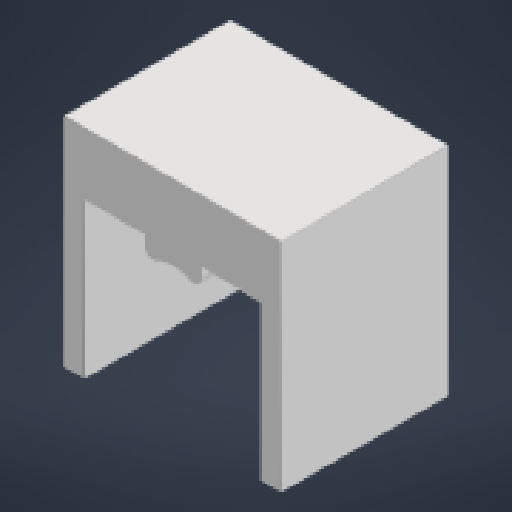
# Autodesk Inventor part: PRINTED resin filament path
Saved by Autodesk Inventor 2024 (Build 280153000, 153)
## iProperties
Created: 2024-07-28
Part Number: PRINTED resin filament path
Material: Generic
Document SubType Name: Modeling
Designer: mateu
Density: 1 g/cm^3
Appearance: Default
Author: mateu
Autodesk Inventor part; units mm, degrees
ref_plane "YZ Plane" through (0, 0, 0) normal (1, 0, 0) x (0, 1, 0)
ref_plane "XZ Plane" through (0, 0, 0) normal (0, 1, 0) x (-1, 0, 0)
ref_plane "XY Plane" through (0, 0, 0) normal (0, 0, 1) x (1, 0, 0)
sketch "Sketch1" plane through (0, 0, 0) normal (0, 0, 1) x (1, 0, 0)
  line L0 (3.45, 2.4) -> (3.45, 4.7)
  line L1 (3.45, 4.7) -> (1.9, 4.7)
  line L2 (1.9, 2.4) -> (1.9, 4.7)
  line L3 (0, 2.4) -> (0, 4.7)
  line L4 (0, 4.7) -> (-1.55, 4.7)
  line L5 (-1.55, 2.4) -> (-1.55, 4.7)
  line L6 (-1.55, 0) -> (-1.55, 2.4)
  line L7 (3.45, 0) -> (3.45, 2.4)
  circle A0 centre (0.95, 3.425) radius 1
  line L8 (4.45, -0.05) -> (4.45, 6.95)
  line L9 (4.45, 6.95) -> (-2.55, 6.95)
  line L10 (-2.55, -0.05) -> (-2.55, 6.95)
  line L11 (-2.25, 6.65) -> (4.15, 6.65)
  line L12 (4.15, 6.65) -> (4.15, 0.25)
  line L13 (4.15, 0.25) -> (-2.25, 0.25)
  line L14 (-2.25, 0.25) -> (-2.25, 6.65)
  line L15 (1.8, 2.4) -> (1.8, 4.8)
  line L16 (1.8, 4.8) -> (3.55, 4.8)
  line L17 (3.55, 4.8) -> (3.55, 2.4)
  line L18 (3.55, 2.4) -> (3.55, 0)
  line L19 (-1.65, 0) -> (-1.65, 2.4)
  line L20 (-1.65, 2.4) -> (-1.65, 4.8)
  line L21 (-1.65, 4.8) -> (0.1, 4.8)
  line L22 (0.1, 4.8) -> (0.1, 2.4)
  circle A1 centre (0.95, 3.425) radius 0.875
  circle A2 centre (0.95, 3.425) radius 1
  circle A3 centre (1.55, 4.521586) radius 0.25
  circle A4 centre (0.35, 4.521586) radius 0.25
  line L23 (4.45, -0.05) -> (-2.55, -0.05)
  point P0 (0, 0)
  point P1 (-1.65, 0.25)
  point P2 (0.1, 4.521586)
  point P3 (0.47, 4.302268)
  point P4 (1.43, 4.302268)
  point P5 (1.8, 4.521586)
  point P6 (3.55, 0.25)
  dimension "d0" = 0.3
  dimension "d1" = 0.1
  dimension "d2" = 0.1
  dimension "d3" = 2
  dimension "d4" = 0.5
  constraints: 24 end point, 4 tangent, 3 centre point, 1 coincident, 1 equal radius, 7 other
  measures "d0" distance between parallel lines of L9 L11
  measures "d1" distance between parallel lines of L0 L17
  measures "d2" distance between parallel lines of L4 L21
  measures "d3" diameter of A2
  measures "d4" diameter of A3
extrude "Extrusion1" add sketch "Sketch1" against normal blind 4.9 contours L18 L17 L16 L15 A3 A0 A4 L22 L21 L20 L19 L13 L14 L11 L12 | A3 | A4
sketch "Sketch2" plane through (0, 0, -4.9) normal (0, 0, -1) x (-1, 0, 0)
  line L0 (-3.55, 0.25) -> (-4.15, 0.25)
  line L1 (-3.55, 0.25) -> (-3.55, 1.25)
  line L2 (-3.55, 4.8) -> (-3.55, 0.25)
  line L3 (-3.55, 1.25) -> (1.739721, 1.25)
  line L4 (2.25, 6.65) -> (-4.15, 6.65)
  line L5 (-4.15, 6.65) -> (-4.15, 0.25)
  line L6 (-4.15, 0.25) -> (-3.55, 0.25)
  line L7 (-3.55, 0.25) -> (-3.55, 4.8)
  line L8 (-3.55, 4.8) -> (-1.8, 4.8)
  line L9 (-1.8, 4.8) -> (-1.8, 4.521586)
  arc A0 (-1.8, 4.521586) -> (-1.43, 4.302268) centre (-1.55, 4.521586) ccw
  arc A1 (-0.47, 4.302268) -> (-1.43, 4.302268) centre (-0.95, 3.425) ccw
  arc A2 (-0.47, 4.302268) -> (-0.1, 4.521586) centre (-0.35, 4.521586) ccw
  line L10 (-0.1, 4.521586) -> (-0.1, 4.8)
  line L11 (-0.1, 4.8) -> (1.65, 4.8)
  line L12 (1.65, 4.8) -> (1.65, 0.25)
  line L13 (1.65, 0.25) -> (2.25, 0.25)
  line L14 (2.25, 0.25) -> (2.25, 6.65)
  circle A3 centre (-0.95, 3.425) radius 1
  point P0 (0, 0)
  point P1 (1.65, 1.25)
  point P2 (-0.47, 4.302268)
  dimension "d8" = 1
  constraints: 4 end point, 1 centre point, 1 coincident, 1 concentric, 1 perpendicular, 1 point on line
  measures "d8" distance of L0.start L1.end
extrude "Extrusion2" add sketch "Sketch2" against normal blind 0.8 contours L2 L8 L9 A0 A3 A2 L10 L11 L12 L3
chamfer "Chamfer1" distance 0.5 angle 20 1 edges at (0.95, 2.425, -4.1) measured on face at (0.95, 2.425, -4.6)
sketch "Sketch3" plane through (0, 0, 0) normal (0, 0, 1) x (1, 0, 0)
  arc A0 (0.189544, 4.329873) -> (1.710456, 4.329873) centre (0.95, 3.425) ccw
  arc A1 (0.1, 4.521586) -> (0.189544, 4.329873) centre (0.35, 4.521586) ccw
  line L0 (0.1, 4.8) -> (0.1, 4.521586)
  line L1 (-1.65, 4.8) -> (0.1, 4.8)
  line L2 (-1.65, 1.25) -> (-1.65, 4.8)
  line L3 (-1.65, 1.25) -> (3.55, 1.25)
  line L4 (3.55, 4.8) -> (3.55, 1.25)
  line L5 (1.8, 4.8) -> (3.55, 4.8)
  line L6 (1.8, 4.521586) -> (1.8, 4.8)
  arc A2 (1.710456, 4.329873) -> (1.8, 4.521586) centre (1.55, 4.521586) ccw
  spline S0 degree 7 poles (1.710456, 4.329873) (1.702909, 4.323556) (1.695037, 4.317557) (1.686841, 4.311886) (1.678321, 4.306557) (1.669477, 4.301587) (1.660303, 4.296994) (1.636622, 4.286561) (1.621727, 4.281222) (1.606064, 4.276852) (1.589598, 4.273563) (1.572312, 4.271515) (1.554218, 4.270908) (1.520976, 4.272859) (1.506137, 4.274699) (1.490907, 4.277659) (1.475421, 4.281858) (1.459899, 4.287391) (1.444641, 4.294258) (1.43, 4.302268) knots 0 0 0 0 0 0 0 0 0.27575999 0.27575999 0.27575999 0.27575999 0.27575999 0.27575999 0.6867657 0.6867657 0.6867657 0.6867657 0.6867657 0.6867657 1 1 1 1 1 1 1 1
  arc A3 (0.47, 4.302268) -> (1.43, 4.302268) centre (0.95, 3.425) ccw
  spline S1 degree 7 poles (0.47, 4.302268) (0.46268, 4.298263) (0.455202, 4.294542) (0.44761, 4.291129) (0.439944, 4.288037) (0.432244, 4.28527) (0.424545, 4.282826) (0.412361, 4.279443) (0.407854, 4.278298) (0.403363, 4.277261) (0.398893, 4.276329) (0.394447, 4.2755) (0.390029, 4.274771) (0.373693, 4.272418) (0.361978, 4.271418) (0.350539, 4.271076) (0.339399, 4.271331) (0.328568, 4.272128) (0.318044, 4.273419) (0.287546, 4.27864) (0.268478, 4.283907) (0.250537, 4.290674) (0.233693, 4.298769) (0.217921, 4.308053) (0.203205, 4.318439) (0.189544, 4.329873) knots 0 0 0 0 0 0 0 0 0.1568747 0.1568747 0.1568747 0.1568747 0.1568747 0.1568747 0.24930104 0.24930104 0.24930104 0.24930104 0.24930104 0.24930104 0.50102336 0.50102336 0.50102336 0.50102336 0.50102336 0.50102336 1 1 1 1 1 1 1 1
  arc A4 (0.189544, 4.329873) -> (1.710456, 4.329873) centre (0.95, 3.425) ccw
  point P0 (0, 0)
  point P1 (1.710456, 4.329873)
  point P2 (0.189544, 4.329873)
  constraints: 2 other
extrude "Extrusion3" add sketch "Sketch3" against normal blind 0.9
chamfer "Chamfer2" distance 0.5 angle 20 2 edges at (0.95, 4.425, 0) (0.95, 2.425, 0) measured on face at (0.95, 4.425, -0.5) measured on face at (0.95, 2.425, -0.5)
body "Solid1"
